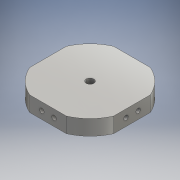
# Autodesk Inventor part: Bottom
Saved by Autodesk Inventor 2016 (Build 200138000, 138)
## iProperties
Created: 2016-06-22
Part Number: Bottom
Material: Generic
Document SubType Name: Modeling
Designer: Andres
Density: 1 g/cm^3
Appearance: Aluminum - Polished
Author: Andres
Autodesk Inventor part; units mm, degrees
ref_plane "YZ Plane" through (0, 0, 0) normal (1, 0, 0) x (0, 1, 0)
ref_plane "XZ Plane" through (0, 0, 0) normal (0, 1, 0) x (-1, 0, 0)
ref_plane "XY Plane" through (0, 0, 0) normal (0, 0, 1) x (1, 0, 0)
sketch "Sketch1" plane through (0, 0, 0) normal (0, 0, 1) x (1, 0, 0)
  circle A0 centre (0, 0) radius 30
  dimension "d0" = 60
  constraints: 1 centre point, 1 coincident
  measures "d0" diameter of A0
extrude "Extrusion1" add sketch "Sketch1" along normal blind 10
sketch "Sketch2" plane through (0, 0, 10) normal (0, 0, 1) x (1, 0, 0)
  line L0 (-27.5, -27.5) -> (27.5, -27.5)
  line L1 (27.5, -27.5) -> (27.5, 27.5)
  line L2 (27.5, 27.5) -> (-27.5, 27.5)
  line L3 (-27.5, 27.5) -> (-27.5, -27.5)
  line L4 (-27.5, -27.5) -> (27.5, 27.5) construction
  line L5 (27.5, -27.5) -> (-27.5, 27.5) construction
  point P0 (0, 0)
  dimension "d3" = 55
  dimension "d4" = 55
  constraints: 12 end point, 2 midpoint, 2 parallel, 1 horizontal, 1 perpendicular
  measures "d3" distance of L2.end L1.end
  measures "d4" distance of L1.end L0.end
extrude "Extrusion2" cut sketch "Sketch2" against normal blind 10 keep common part
sketch "Sketch3" plane through (-27.5, -11.9896, 10) normal (-1, 0, 0) x (0, 0, 1)
  point P0 (-10, 11.9896)
sketch "Sketch4" plane through (0, 0, 10) normal (0, 0, 1) x (1, 0, 0)
  circle A0 centre (0, 0) radius 2.5
  dimension "d7" = 5
  constraints: 1 centre point, 1 coincident
  measures "d7" diameter of A0
extrude "Extrusion3" cut sketch "Sketch4" against normal blind 10
sketch "Sketch5" plane through (-11.9896, -27.5, 10) normal (0, -1, 0) x (1, 0, 0)
  circle A0 centre (7.9896, -5) radius 1.5
  circle A1 centre (15.9896, -5) radius 1.5
  line L0 (23.9792, 0) -> (0, 0) projected
  line L1 (0, 0) -> (0, -10) projected
  point P0 (11.9896, -10)
  dimension "d10" = 3
  dimension "d11" = 3
  dimension "d12" = 8
  dimension "d13" = 5
  dimension "d14" = 5
  dimension "d15" = 7.9896
  constraints: 2 centre point
  measures "d10" diameter of A0
  measures "d11" diameter of A1
  measures "d12" distance of A1.centre A0.centre
  measures "d13" distance from line of L0 A1.centre
  measures "d14" distance from line of L0 A0.centre
  measures "d15" distance from line of L1 A0.centre
sketch "Sketch6" plane through (27.5, -11.9896, 10) normal (1, 0, 0) x (0, 0, -1)
  circle A0 centre (5, 7.9896) radius 1.5
  circle A1 centre (5, 15.9896) radius 1.5
  line L0 (0, 23.9792) -> (0, 0) projected
  line L1 (0, 0) -> (10, 0) projected
  point P0 (10, 11.9896)
  dimension "d16" = 3
  dimension "d17" = 3
  dimension "d18" = 8
  dimension "d19" = 5
  dimension "d20" = 5
  dimension "d21" = 7.9896
  constraints: 2 centre point
  measures "d16" diameter of A0
  measures "d17" diameter of A1
  measures "d18" distance of A1.centre A0.centre
  measures "d19" distance from line of L0 A0.centre
  measures "d20" distance from line of L0 A1.centre
  measures "d21" distance from line of L1 A0.centre
sketch "Sketch7" plane through (-11.9896, 27.5, 10) normal (0, 1, 0) x (1, 0, 0)
  circle A0 centre (15.9896, 5) radius 1.5
  circle A1 centre (7.9896, 5) radius 1.5
  line L0 (0, 0) -> (0, 10) projected
  line L1 (0, 0) -> (23.9792, 0) projected
  point P0 (11.9896, 10)
  dimension "d22" = 3
  dimension "d23" = 3
  dimension "d24" = 8
  dimension "d25" = 7.9896
  dimension "d26" = 5
  dimension "d27" = 5
  constraints: 2 centre point
  measures "d22" diameter of A0
  measures "d23" diameter of A1
  measures "d24" distance of A1.centre A0.centre
  measures "d25" distance from line of L0 A1.centre
  measures "d26" distance from line of L1 A1.centre
  measures "d27" distance from line of L1 A0.centre
sketch "Sketch8" plane through (-27.5, -11.9896, 10) normal (-1, 0, 0) x (0, 0, 1)
  circle A0 centre (-5, 15.9896) radius 1.5
  circle A1 centre (-5, 7.9896) radius 1.5
  line L0 (0, 23.9792) -> (-10, 23.9792) projected
  line L1 (0, 0) -> (0, 23.9792) projected
  point P0 (-10, 11.9896)
  dimension "d28" = 3
  dimension "d29" = 3
  dimension "d30" = 7.9896
  dimension "d31" = 5
  dimension "d32" = 5
  dimension "d33" = 8
  constraints: 2 centre point
  measures "d28" diameter of A0
  measures "d29" diameter of A1
  measures "d30" distance from line of L0 A0.centre
  measures "d31" distance from line of L1 A1.centre
  measures "d32" distance from line of L1 A0.centre
  measures "d33" distance of A1.centre A0.centre
extrude "Extrusion4" cut sketch "Sketch6" against normal blind 20
extrude "Extrusion5" cut sketch "Sketch7" against normal blind 20
extrude "Extrusion6" cut sketch "Sketch8" against normal blind 20
extrude "Extrusion7" cut sketch "Sketch5" against normal blind 20
body "Solid1"
